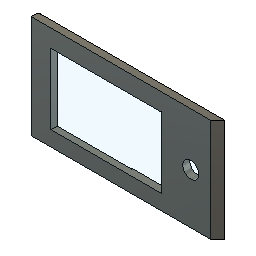
LRF Window Frame v6 (Autodesk Fusion 360 design; units mm, degrees)
Autodesk Fusion 360 part; units mm, degrees
sketch "Sketch1" plane through (0, 0, 0) normal (0, 0, 1) x (1, 0, 0)
  line L0 (0, 0) -> (45.4152, 0)
  line L1 (45.4152, 0) -> (45.4152, 26.035)
  line L2 (45.4152, 26.035) -> (0, 26.035)
  line L3 (0, 26.035) -> (0, 0)
  line L4 (5.0292, 21.59) -> (32.893, 21.59)
  line L5 (32.893, 21.59) -> (32.893, 3.81)
  line L6 (32.893, 3.81) -> (5.0292, 3.81)
  line L7 (5.0292, 3.81) -> (5.0292, 21.59)
  circle A0 centre (40.3352, 12.7) radius 2.032
  dimension "d1" = 45.4152
  dimension "d2" = 26.035
  dimension "d3" = 27.8638
  dimension "d4" = 17.78
  dimension "d5" = 5.0292
  dimension "d6" = 3.81
  dimension "d7" = 4.064
  dimension "d8" = 5.08
  dimension "d9" = 12.7
  constraint horizontal L0
  constraint vertical L1
  constraint horizontal L2
  constraint vertical L3
  constraint coincident L0.start L3.end
  constraint horizontal L4
  constraint vertical L5
  constraint horizontal L6
  constraint vertical L7
  measures "d1" distance of L0.start L0.end
  measures "d2" distance of L0.start L2.end
  measures "d3" distance of L4.start L4.end
  measures "d4" distance of L4.start L6.end
  measures "d5" distance of L3 L7
  measures "d6" distance of L0 L6
  measures "d7" diameter of A0
  measures "d8" distance of L1 A0.centre
  measures "d9" distance of L0 A0.centre
extrude "Extrude1" add sketch "Sketch1" along normal blind 1.778
sketch "Sketch2" plane through (0, 0, 0) normal (0, 0, -1) x (-1, 0, 0)
  line L0 (-5.0292, 3.81) -> (-32.893, 3.81)
  line L1 (-32.893, 3.81) -> (-32.893, 21.59)
  line L2 (-32.893, 21.59) -> (-5.0292, 21.59)
  line L3 (-5.0292, 21.59) -> (-5.0292, 3.81)
  circle A0 centre (-40.3352, 12.7) radius 2.032
  line L4 (0, 0) -> (0, 26.035)
  line L5 (0, 26.035) -> (-45.4152, 26.035)
  line L6 (-45.4152, 26.035) -> (-45.4152, 0)
  line L7 (-45.4152, 0) -> (0, 0)
  line L8 (-2.9972, 0) -> (-23.8252, 0)
  line L9 (-23.8252, 0) -> (-23.8252, 23.876)
  line L10 (-23.8252, 23.876) -> (-2.9972, 23.876)
  line L11 (-2.9972, 23.876) -> (-2.9972, 0)
  line L12 (-2.9972, 23.876) -> (-2.9972, 26.035)
  dimension "d12" = 20.828
  dimension "d13" = 23.876
  dimension "d14" = 2.9972
  constraint horizontal L8
  constraint vertical L9
  constraint horizontal L10
  constraint vertical L11
  constraint coincident L7 L8.start
  constraint coincident L5 L12.end
  constraint perpendicular L5 L12
  measures "d12" distance of L8.start L8.end
  measures "d13" distance of L8.start L10.end
  measures "d14" distance of L4 L11
extrude "Extrude2" cut sketch "Sketch2" against normal blind 0.2032 contours L0 L2 L3 L7 L8 L9 L10 L11
sketch "Sketch3" plane through (0, 0, 1.778) normal (0, 0, 1) x (1, 0, 0)
  line L0 (32.893, 3.81) -> (5.0292, 3.81)
  line L1 (5.0292, 3.81) -> (5.0292, 21.59)
  line L2 (5.0292, 21.59) -> (32.893, 21.59)
  line L3 (32.893, 21.59) -> (32.893, 3.81)
  circle A0 centre (40.3352, 12.7) radius 2.032
  line L4 (0, 26.035) -> (0, 0)
  line L5 (0, 0) -> (45.4152, 0)
  line L6 (45.4152, 0) -> (45.4152, 26.035)
  line L7 (45.4152, 26.035) -> (0, 26.035)
fillet "Fillet1" radius 0.635 1 edges at (0, 13.0175, 0)
draft "Draft1" angle 45 neutral plane through (0, 0, 1.778) pull (0, 0, 1) 1 faces at (45.4152, 17.3567, 0.5927)
